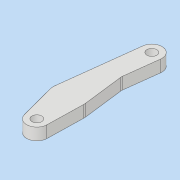
# Autodesk Inventor part: CarrageRodEndMount
Saved by Autodesk Inventor 2017 (Build 210142000, 142)
## iProperties
Created: 2018-04-09
Part Number: CarrageRodEndMount
Material: ABS Plastic
Document SubType Name: Modeling
Designer: Derek Wider
Density: 1.06 g/cm^3
Appearance: Smooth - White
Author: Derek Wider
Autodesk Inventor part; units mm, degrees
ref_plane "YZ Plane" through (0, 0, 0) normal (1, 0, 0) x (0, 1, 0)
ref_plane "XZ Plane" through (0, 0, 0) normal (0, 1, 0) x (-1, 0, 0)
ref_plane "XY Plane" through (0, 0, 0) normal (0, 0, 1) x (1, 0, 0)
sketch "Sketch1" plane through (0, 0, 0) normal (0, 1, 0) x (-1, 0, 0)
  circle A0 centre (0, 0) radius 1.8415
  circle A1 centre (0, -42.8625) radius 1.8415
  line L0 (0, 0) -> (0, -42.8625) construction
  circle A2 centre (1.615, -13.4938) radius 3.3655
  circle A3 centre (1.615, -29.3687) radius 1.7145
  line L1 (1.615, -29.3687) -> (1.615, -13.4938) construction
  circle A4 centre (0, 0) radius 3.81
  circle A5 centre (0, -42.8625) radius 3.81
  circle A6 centre (1.615, -13.4938) radius 5.715
  circle A7 centre (1.615, -29.3687) radius 3.81
  line L2 (7.1383, -12.0259) -> (3.6822, 0.9786)
  line L3 (-3.8091, 0.082) -> (-4.0987, -13.3708)
  line L4 (-4.0575, -14.1898) -> (-2.195, -29.3687)
  line L5 (7.2887, -14.1796) -> (5.3975, -29.826)
  line L6 (3.783, -43.3153) -> (5.3975, -29.826)
  line L7 (-3.7821, -42.402) -> (-2.195, -29.3687)
  point P0 (-37.12, -21.4312)
  point P1 (0, -21.4312)
  point P2 (1.615, -21.4312)
  dimension "d0" = 3.683
  dimension "d1" = 42.8625
  dimension "d2" = 42.8625
  dimension "d3" = 6.731
  dimension "d4" = 3.429
  dimension "d5" = 15.875
  dimension "d6" = 38.735
  dimension "d7" = 7.62
  dimension "d8" = 11.43
  dimension "d9" = 7.62
  constraints: 16 end point, 10 point on circle, 8 centre point, 8 tangent, 5 coincident, 2 equal radius, 2 horizontal alignment, 2 midpoint, 2 vertical, 1 vertical alignment
  measures "d0" diameter of A0
  measures "d1" distance of L0.end point (0, 0)
  measures "d2" distance of point (-37.12, -21.431) point (0, 0)
  measures "d3" diameter of A2
  measures "d4" diameter of A3
  measures "d5" distance of L1.end L1.start
  measures "d6" distance of point (-37.12, -21.431) point (1.615, -21.431)
  measures "d7" diameter of A4
  measures "d8" diameter of A6
  measures "d9" diameter of A7
extrude "Extrusion1" add sketch "Sketch1" along normal blind 3.175
sketch "Sketch2" plane through (0, 3.175, 0) normal (0, 1, 0) x (1, 0, 0)
  circle A0 centre (-1.615, 13.4938) radius 3.3655 projected
  circle A1 centre (0, 0) radius 1.8415 projected
  circle A2 centre (-1.615, 29.3687) radius 1.7145 projected
  circle A3 centre (0, 42.8625) radius 1.8415 projected
  arc A4 (3.7821, 42.402) -> (-3.783, 43.3153) centre (0, 42.8625) ccw projected
  line L0 (-3.783, 43.3153) -> (-5.3975, 29.826) projected
  line L1 (-5.3975, 29.826) -> (-7.2887, 14.1796) projected
  arc A5 (-7.2887, 14.1796) -> (-7.1383, 12.0259) centre (-1.615, 13.4938) ccw projected
  line L2 (-7.1383, 12.0259) -> (-3.6822, -0.9786) projected
  arc A6 (-3.6822, -0.9786) -> (3.8091, -0.082) centre (0, 0) ccw projected
  line L3 (3.8091, -0.082) -> (4.0987, 13.3708) projected
  arc A7 (4.0987, 13.3708) -> (4.0575, 14.1898) centre (-1.615, 13.4938) ccw projected
  line L4 (4.0575, 14.1898) -> (2.195, 29.3687) projected
  line L5 (2.195, 29.3687) -> (3.7821, 42.402) projected
  point P0 (0, 0)
extrude "Extrusion2" add sketch "Sketch2" along normal blind 1.27 contours A0 | A2 | L5 L4 A7 L3 A6 L2 A5 L1 L0 A4
fillet "Fillet1" radius 3.175 1 edges at (2.195, 2.2225, -29.3687)
body "Solid1"
